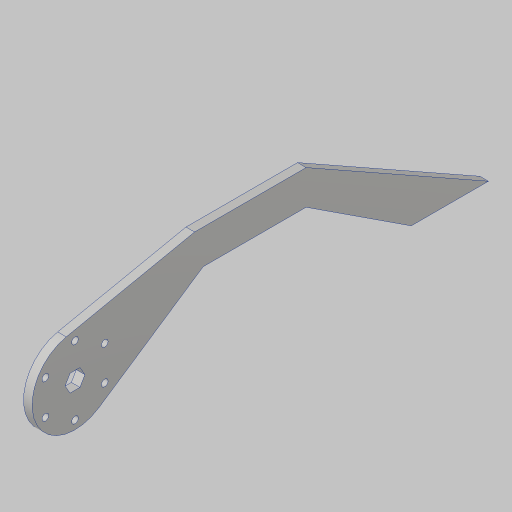
# Autodesk Inventor part: CL4-025
Saved by Autodesk Inventor 2023.5 (Build 275446000, 446)
## iProperties
Created: 2025-02-13
Part Number: CL4-025
Material: Aluminum 6061
Document SubType Name: Modeling
Designer: slick
Density: 2.7 g/cm^3
Appearance: Aluminum - Flat
Author: slick
Autodesk Inventor part; units mm, degrees
ref_plane "YZ Plane" through (0, 0, 0) normal (1, 0, 0) x (0, 1, 0)
ref_plane "XZ Plane" through (0, 0, 0) normal (0, 1, 0) x (-1, 0, 0)
ref_plane "XY Plane" through (0, 0, 0) normal (0, 0, 1) x (1, 0, 0)
sketch "Sketch1" plane through (0, 0, 0) normal (1, 0, 0) x (0, 1, 0)
  circle A0 centre (0, 0) radius 31.75 construction
  line L0 (19.05, -103.6647) -> (-107.95, -103.6647) construction
  line L1 (-107.95, -103.6647) -> (-107.95, -162.179) construction
  line L2 (-107.95, -162.179) -> (19.05, -162.179) construction
  line L3 (19.05, -162.179) -> (19.05, -103.6647) construction
  line L4 (19.05, -103.6647) -> (-107.95, -162.179) construction
  line L5 (-107.95, -103.6647) -> (19.05, -162.179) construction
  line L6 (-25.4, -162.179) -> (-25.4, -365.379) construction
  point P0 (-44.45, -132.9219)
  dimension "d0" = 63.5
  dimension "d2" = 127
  dimension "d3" = 58.5143
  dimension "d4" = 19.05
  dimension "d5" = 162.179
  dimension "d6" = 203.2
  dimension "d7" = 25.4
  constraints: 14 end point, 2 midpoint, 2 parallel, 1 centre point, 1 coincident, 1 horizontal, 1 perpendicular, 1 point on line, 1 vertical
  measures "d0" diameter of A0
  measures "d2" distance of L1.end L2.end
  measures "d3" distance of L2.end L0.start
  measures "d4" horizontal distance of L0.start point (0, 0)
  measures "d5" distance from line of L2 point (0, 0)
  measures "d6" distance of L6.start L6.end
  measures "d7" distance from line of L6 point (0, 0)
sketch "Sketch2" plane through (0, 0, 0) normal (1, 0, 0) x (0, 1, 0)
  circle A0 centre (0, 0) radius 31.75 construction
  line L0 (19.05, -103.6647) -> (-107.95, -103.6647) construction
  line L1 (-107.95, -103.6647) -> (-107.95, -162.179) construction
  line L2 (-107.95, -162.179) -> (19.05, -162.179) construction
  line L3 (19.05, -162.179) -> (19.05, -103.6647) construction
  line L4 (19.05, -103.6647) -> (-107.95, -162.179) construction
  line L5 (-107.95, -103.6647) -> (19.05, -162.179) construction
  line L6 (-25.4, -162.179) -> (-25.4, -365.379) construction
  line L7 (-26.3632, -17.693) -> (25.4, -94.8219)
  line L8 (25.4, -94.8219) -> (25.4, -171.0219)
  line L9 (25.4, -171.0219) -> (-25.4, -248.7885)
  line L10 (31.0868, 6.4557) -> (50.8, -88.4719)
  line L11 (50.8, -88.4719) -> (50.8, -171.0219)
  line L12 (50.8, -171.0219) -> (-25.4, -305.9385)
  arc A1 (31.0868, 6.4557) -> (-26.3632, -17.693) centre (0, 0) ccw
  line L13 (6.35, 3.6662) -> (6.35, -3.6662)
  line L14 (6.35, -3.6662) -> (0, -7.3323)
  line L15 (0, -7.3323) -> (-6.35, -3.6662)
  line L16 (-6.35, -3.6662) -> (-6.35, 3.6662)
  line L17 (-6.35, 3.6662) -> (0, 7.3323)
  line L18 (0, 7.3323) -> (6.35, 3.6662)
  line L19 (-25.4, -248.7885) -> (-25.4, -305.9385)
  point P0 (-44.45, -132.9219)
  point P1 (25.4, -132.9219)
  point P2 (19.05, -132.9219)
  point P3 (-6.35, 0)
  dimension "d8" = 6.35
  dimension "d9" = 76.2
  dimension "d10" = 25.4
  dimension "d11" = 82.55
  dimension "d12" = 12.7
  dimension "d13" = 57.15
  constraints: 26 end point, 4 point on circle, 3 midpoint, 3 vertical, 2 coincident, 2 horizontal alignment, 2 point on line, 2 tangent, 1 centre point, 1 equal length, 13 other
  measures "d8" distance between parallel lines of L3 L8
  measures "d9" distance of L7.end L8.end
  measures "d10" distance between parallel lines of L8 L11
  measures "d11" distance of L10.end L11.end
  measures "d12" distance from line of point (-6.35, 0) L13
  measures "d13" distance of L12.end L9.end
extrude "Extrusion1" add sketch "Sketch2" along normal blind 6.35
sketch "Sketch3" plane through (6.35, 0, 0) normal (1, 0, 0) x (0, 0, -1)
  circle A0 centre (0, 0) radius 25.4 construction
  point P0 (0, 25.4)
  point P1 (-21.997, 12.7)
  point P2 (-21.997, -12.7)
  point P3 (0, -25.4)
  point P4 (21.997, -12.7)
  point P5 (21.997, 12.7)
  dimension "d16" = 50.8
  dimension "d19" = 360
  constraints: 2 vertical alignment, 1 coincident, 9 other
hole "Hole1" at (6.35, 25.4, 0) at (6.35, 12.7, 21.997) at (6.35, -12.7, 21.997) at (6.35, -25.4, 0) at (6.35, -12.7, -21.997) at (6.35, 12.7, -21.997) direction (-1, 0, 0) diameter 5.1054 end through all clearance for "Flat Head Machine Screw (82)" size "#10" standard "Ansi Unified Screw Threads"
body "Solid1"
